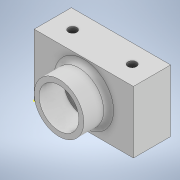
# Autodesk Inventor part: charging_port
Saved by Autodesk Inventor 2021 (Build 250183000, 183)
## iProperties
Created: 2020-11-14
Part Number: charging_port
Material: Generic
Document SubType Name: Modeling
Designer: elizabethhassan
Density: 1 g/cm^3
Appearance: Default
Author: elizabethhassan
Autodesk Inventor part; units mm, degrees
ref_plane "YZ Plane" through (0, 0, 0) normal (1, 0, 0) x (0, 1, 0)
ref_plane "XZ Plane" through (0, 0, 0) normal (0, 1, 0) x (-1, 0, 0)
ref_plane "XY Plane" through (0, 0, 0) normal (0, 0, 1) x (1, 0, 0)
sketch "Sketch1" plane through (0, 0, 0) normal (0, 0, 1) x (1, 0, 0)
  line L0 (0, 0) -> (40, 0)
  line L1 (40, 0) -> (40, 25)
  line L2 (40, 25) -> (0, 25)
  line L3 (0, 25) -> (0, 0)
  dimension "d0" = 40
  dimension "d1" = 25
  constraints: 8 end point, 2 parallel, 1 horizontal, 1 perpendicular
  measures "d0" distance of L2.end L1.end
  measures "d1" distance of L1.end L0.end
extrude "Extrusion1" add sketch "Sketch1" along normal blind 15
sketch "Sketch2" plane through (0, 25, 0) normal (0, 1, 0) x (1, 0, 0)
  line L0 (0, 0) -> (0, -15) projected
  line L1 (0, -7.5) -> (8, -7.5)
  line L2 (40, 0) -> (40, -15) projected
  line L3 (40, -7.5) -> (32, -7.5)
  dimension "d4" = 8
  dimension "d5" = 8
  constraints: 4 end point, 2 horizontal, 2 midpoint
  measures "d4" distance of L1.start L1.end
  measures "d5" distance of L3.start L3.end
hole "Hole1" at (8, 25, 7.5) at (32, 25, 7.5) direction (0, -1, 0) diameter 3.4587 depth 10.8 tip angle 118 thread size "M4x0.5" class "6H" standard "ANSI Metric M Profile"
sketch "Sketch3" plane through (0, 0, 15) normal (0, 0, 1) x (1, 0, 0)
  line L0 (40, 25) -> (0, 25) projected
  line L1 (20, 25) -> (20, 0) construction
  line L2 (0, 0) -> (40, 0) projected
  circle A0 centre (20, 12.5) radius 10
  circle A1 centre (20, 12.5) radius 8
  dimension "d13" = 20
  constraints: 3 midpoint, 2 centre point, 2 end point
  measures "d13" diameter of A0
extrude "Extrusion2" add sketch "Sketch3" along normal blind 10
sketch "Sketch4" plane through (0, 0, 0) normal (0, -1, 0) x (1, 0, 0)
  line L0 (0, 15) -> (40, 15) projected
  line L1 (20, 15) -> (20, 0)
  line L2 (40, 0) -> (0, 0) projected
  point P0 (20, 7.5)
  constraints: 3 midpoint, 2 end point
hole "Hole2" at (20, 0, 7.5) direction (0, 1, 0) diameter 3.4587 depth 10.8 tip angle 118 thread size "M4x0.5" class "6H" standard "ANSI Metric M Profile"
fillet "Fillet1" radius 2 1 edges at (10, 12.5, 15)
sketch "Sketch5" plane through (20, 12.5, 15) normal (0, 0, 1) x (1, 0, 0)
  point P0 (-20, -12.5)
body "Solid1"
